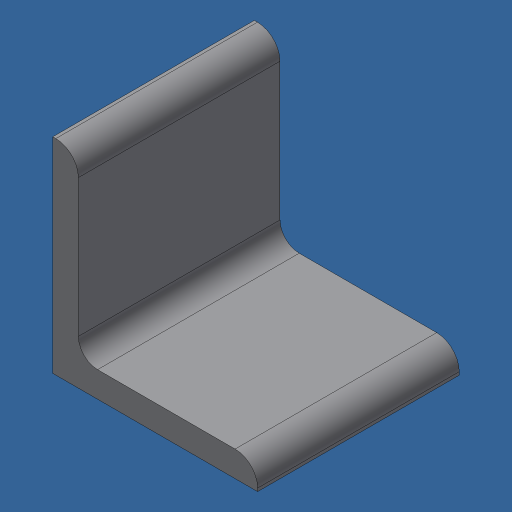
# Autodesk Inventor part: ANGLE IRON, 4 X 4 X 0.50 THK
Saved by Autodesk Inventor 2024.3 (Build 283343000, 343)
## iProperties
Category: _
Manager: _
Created: 2023-11-08
Part Number: ANGLE IRON, 4 X 4 X 0.50 THK
Checked By: 00
Engr Approved By: _
User Status: Work In Process
Material: Angle Iron
Description: ANGLE IRON, 4 X 4 X 0.50 THK
Document SubType Name: Modeling
Mfg Approved By: Stephen.Oerton
Designer: -
Mass: 1874.78 g
Surface Area: 440.422 cm^2
Volume: 238.521 cm^3
Density: 7.86 g/cm^3
Appearance: Grey (Light)
ILogicPurgeVersion: 2.2.20.20
OnSaveVersion: 2.2.20.20
CN_MASS: 1.87
CN_SERVICEABLE: _
CL_runCount: 0
FIRST_DESCRIPTION: _
SECOND_DESCRIPTION: _
THIRD_DESCRIPTION: _
ModelCat: Uncategorized
Subject: _
Author: -
Keywords: -
Revision Number: A
Autodesk Inventor part; units mm, degrees
ref_plane "YZ Plane" through (0, 0, 0) normal (1, 0, 0) x (0, 1, 0)
ref_plane "XZ Plane" through (0, 0, 0) normal (0, 1, 0) x (-1, 0, 0)
ref_plane "XY Plane" through (0, 0, 0) normal (0, 0, 1) x (1, 0, 0)
sketch "Sketch1" plane through (0, 0, 0) normal (0, 0, 1) x (1, 0, 0)
  line L0 (0, 0) -> (0, 101.6)
  line L1 (0, 101.6) -> (1.524, 101.6)
  line L2 (12.7, 90.424) -> (12.7, 22.225)
  line L3 (0, 0) -> (101.6, 0)
  line L4 (101.6, 0) -> (101.6, 1.524)
  line L5 (90.424, 12.7) -> (22.225, 12.7)
  arc A0 (12.7, 22.225) -> (22.225, 12.7) centre (22.225, 22.225) ccw
  arc A1 (12.7, 90.424) -> (1.524, 101.6) centre (1.524, 90.424) ccw
  arc A2 (101.6, 1.524) -> (90.424, 12.7) centre (90.424, 1.524) ccw
  dimension "thickness" = 12.7
  dimension "d3" = 12.7
  dimension "LegSize" = 101.6
  dimension "d5" = 101.6
  dimension "radius" = 9.525
  dimension "d7" = 11.176
  dimension "d8" = 11.176
  constraints: 12 end point, 6 point on circle, 6 tangent, 4 parallel, 3 centre point, 1 coincident, 1 perpendicular, 1 vertical
  measures "thickness" distance between parallel lines of L2 L0
  measures "d3" distance between parallel lines of L5 L3
  measures "LegSize" distance of L0.start L0.end
  measures "d5" distance of L0.start L3.end
  measures "radius" radius of A0
  measures "d7" radius of A1
  measures "d8" radius of A2
extrude "4\" X 4\" X 1/2\"" add sketch "Sketch1" along normal mid plane 100
equation "\"d3\" = thickness"
equation "\"d5\" = LegSize"
